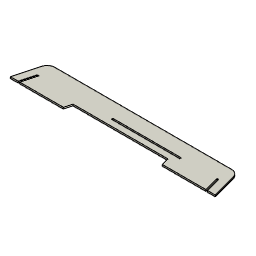
Bar (Autodesk Fusion 360 design; units mm, degrees)
Autodesk Fusion 360 part; units mm, degrees
sketch "Schizzo1" plane through (0, 0, 0) normal (0, 0, 1) x (1, 0, 0)
  line L0 (0, 0) -> (80.3848, 300) construction
  line L1 (80.3848, 300) -> (503.6152, 300) construction
  line L2 (503.6152, 300) -> (584, 0) construction
  line L3 (584, 0) -> (0, 0) construction
  line L4 (53.5898, 200) -> (530.4102, 200) construction
  line L5 (42.8719, 160) -> (541.1281, 160)
  line L6 (64.3078, 240) -> (519.6922, 240)
  line L7 (64.3078, 240) -> (43.6023, 240)
  line L8 (43.6023, 240) -> (22.1663, 160)
  line L9 (22.1663, 160) -> (42.8719, 160)
  line L10 (42.8719, 160) -> (53.5898, 200)
  line L11 (53.5898, 200) -> (57.4204, 200)
  line L12 (57.4204, 200) -> (46.7024, 160)
  line L13 (519.6922, 240) -> (540.3977, 240)
  line L14 (540.3977, 240) -> (561.8337, 160)
  line L15 (561.8337, 160) -> (541.1281, 160)
  line L16 (541.1281, 160) -> (530.4102, 200)
  line L17 (530.4102, 200) -> (526.5796, 200)
  line L18 (526.5796, 200) -> (537.2976, 160)
  line L19 (161.641, 160) -> (167, 180)
  line L20 (167, 180) -> (417, 180)
  line L21 (417, 180) -> (422.359, 160)
  line L22 (292, 180) -> (292, 160) construction
  line L23 (292, 200) -> (252.15, 200)
  line L24 (252.15, 200) -> (252.15, 196.3)
  line L25 (252.15, 196.3) -> (431.85, 196.3)
  line L26 (431.85, 196.3) -> (431.85, 200)
  line L27 (292, 200) -> (431.85, 200)
  dimension "d1" = 75
  dimension "d2" = 75
  dimension "d3" = 584
  dimension "d4" = 300
  dimension "d5" = 200
  dimension "d6" = 40
  dimension "d7" = 40
  dimension "d8" = 3.7
  dimension "d11" = 3.7
  dimension "d12" = 20
  dimension "d13" = 20
  dimension "d14" = 20
  dimension "d15" = 250
  dimension "d20" = 3.7
  dimension "d22" = 139.85
  dimension "d23" = 39.85
  constraint coincident L0.start L3.end
  constraint horizontal L1
  constraint parallel L1 L3
  constraint coincident L0 L4.start
  constraint coincident L2 L4.end
  constraint horizontal L4
  constraint coincident L0 L5.start
  constraint coincident L2 L5.end
  constraint parallel L4 L5
  constraint coincident L0 L6.start
  constraint coincident L2 L6.end
  constraint horizontal L6
  constraint parallel L6 L7
  constraint parallel L0 L8
  constraint parallel L5 L9
  constraint coincident L4 L11.end
  constraint coincident L5 L12.end
  constraint parallel L10 L12
  constraint parallel L6 L13
  constraint coincident L4 L17.end
  constraint coincident L5 L18.end
  constraint parallel L16 L18
  constraint parallel L5 L15
  constraint parallel L2 L14
  constraint coincident L5 L19.start
  constraint parallel L5 L20
  constraint coincident L5 L21.end
  constraint parallel L0 L19
  constraint parallel L2 L21
  constraint midpoint L20 L22.start
  constraint midpoint L5 L22.end
  constraint perpendicular L5 L22
  constraint midpoint L4 L23.start
  constraint coincident L4 L23.end
  constraint parallel L4 L23
  constraint perpendicular L4 L24
  constraint perpendicular L24 L25
  constraint coincident L4 L26.end
  constraint perpendicular L4 L26
  measures "d1" angle of L0 L3
  measures "d2" angle of L2 L3
  measures "d3" distance of L2.end L0.start
  measures "d4" distance of L1 L3
  measures "d5" distance of L3 L4
  measures "d6" distance of L4 L5
  measures "d7" distance of L4 L6
  measures "d8" distance of L10 L12
  measures "d11" distance of L2 L18
  measures "d12" distance of L2 L14
  measures "d13" distance of L0 L8
  measures "d14" distance of L4 L20
  measures "d15" distance of L19.end L20.end
  measures "d20" distance of L23.end L24.end
  measures "d22" distance of L22 L26
  measures "d23" distance of L22 L24
extrude "Estrusione1" add sketch "Schizzo1" along normal blind 4 contours L5 L6 L7 L8 L9 L10 L11 L12 L13 L14 L15 L16 L17 L18 L19 L20 L21
fillet "Raccordo1" radius 20 2 edges at (43.6023, 240, 2) (540.3977, 240, 2)
component "Component" placed x (1, 0, 0) y (0, 1, 0) z (0, 0, 1) at (0, 0, 0)
equation "d8 = h - 2 * t"
equation "h = 4 mm"
equation "t = 0.15 mm"
equation "d11 = h - 2 * t"
equation "d16 = h"
equation "d20 = h - 2 * t"
equation "d22 = 140 mm - t"
equation "d23 = 40 mm - t"
